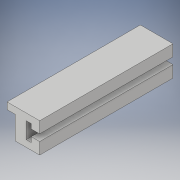
# Autodesk Inventor part: Riel acople de motor
Saved by Autodesk Inventor 2019 (Build 230136000, 136)
## iProperties
Created: 2020-02-02
Part Number: Riel acople de motor
Material: Generic
Document SubType Name: Modeling
Designer: Elías Sánchez
Density: 1 g/cm^3
Appearance: Default
Author: Elías Sánchez
Autodesk Inventor part; units mm, degrees
ref_plane "YZ Plane" through (0, 0, 0) normal (1, 0, 0) x (0, 1, 0)
ref_plane "XZ Plane" through (0, 0, 0) normal (0, 1, 0) x (-1, 0, 0)
ref_plane "XY Plane" through (0, 0, 0) normal (0, 0, 1) x (1, 0, 0)
sketch "Sketch1" plane through (0, 0, 0) normal (0, 0, 1) x (1, 0, 0)
  line L0 (18.475, 5) -> (18.475, -3.5)
  line L1 (18.475, -3.5) -> (12.175, -3.5)
  line L2 (12.175, -12.3) -> (12.175, -8.5)
  line L3 (12.175, -8.5) -> (18.475, -8.5)
  line L4 (18.475, -8.5) -> (18.475, -17.3)
  line L5 (18.475, -17.3) -> (0, -17.3)
  line L6 (0, -17.3) -> (0, 0)
  line L7 (18.475, 5) -> (-6, 5)
  line L8 (-6, 5) -> (-6, 0)
  line L9 (-6, 0) -> (0, 0)
  line L10 (12.175, -3.5) -> (12.175, 0)
  line L11 (12.175, -12.3) -> (8.375, -12.3)
  line L12 (8.375, -12.3) -> (8.375, 0)
  line L13 (8.375, 0) -> (12.175, 0)
  dimension "d0" = 6
  dimension "d1" = 5
  dimension "d2" = 6.3
  dimension "d3" = 6.3
  dimension "d4" = 3.8
  dimension "d6" = 8.375
  dimension "d8" = 5
  dimension "d10" = 5
  dimension "d12" = 3.5
  dimension "d13" = 3.8
  dimension "d14" = 17.3
  constraints: 28 end point, 8 perpendicular, 2 horizontal, 2 point on line, 1 vertical
  measures "d0" distance of L8.end L6.end
  measures "d1" distance of L7.end L8.end
  measures "d2" distance of L0.end L1.end
  measures "d3" distance of L2.end L3.end
  measures "d4" distance between parallel lines of L10 L12
  measures "d6" distance between parallel lines of L6 L12
  measures "d8" distance between parallel lines of L5 L11
  measures "d10" distance between parallel lines of L1 L3
  measures "d12" distance of L1.end L10.end
  measures "d13" distance of L2.start L2.end
  measures "d14" distance between parallel lines of L9 L5
extrude "Extrusion1" add sketch "Sketch1" along normal blind 100
equation "\"d3\" = d2"
equation "\"d13\" = d4"
body "Solid1"
